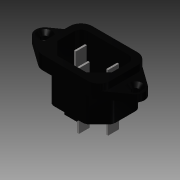
# Autodesk Inventor part: PowerSocket
Saved by Autodesk Inventor 2016 (Build 200138000, 138)
## iProperties
Category: Electronics
Created: 2014-09-28
Part Number: PowerSocket
Material: ABS Plastic
Document SubType Name: Modeling
Designer: Jack
Density: 1.06 g/cm^3
Appearance: Smooth - Black
Mass: 5.27757 g
Surface Area: 54.3399 cm^2
Volume: 4.97884 cm^3
Author: Jack
Title: Power Socket
Autodesk Inventor part; units mm, degrees
ref_plane "YZ Plane" through (0, 0, 0) normal (1, 0, 0) x (0, 1, 0)
ref_plane "XZ Plane" through (0, 0, 0) normal (0, 1, 0) x (-1, 0, 0)
ref_plane "XY Plane" through (0, 0, 0) normal (0, 0, 1) x (1, 0, 0)
sketch "Sketch1" plane through (0, 0, 0) normal (0, 0, 1) x (1, 0, 0)
  circle A0 centre (0, 0) radius 1.6
  circle A1 centre (40, 0) radius 1.6
  circle A2 centre (0, 0) radius 4
  circle A3 centre (40, 0) radius 4
  line L0 (8.5, 11) -> (31.5, 11)
  line L1 (8.5, -11) -> (31.5, -11)
  line L2 (8.5, 11) -> (-2.3275, 3.2531)
  line L3 (-2.3275, -3.2531) -> (8.5, -11)
  line L4 (31.5, -11) -> (42.3275, -3.2531)
  line L5 (42.3275, 3.2531) -> (31.5, 11)
  dimension "d0" = 3.2
  dimension "d2" = 40
  dimension "d3" = 8
  dimension "d5" = 23
  dimension "d6" = 11
  dimension "d7" = 11
  dimension "d8" = 8.5
  constraints: 12 end point, 4 centre point, 4 point on circle, 4 tangent, 3 coincident, 2 equal radius, 2 horizontal, 1 horizontal alignment, 1 parallel, 1 vertical alignment
  measures "d0" diameter of A0
  measures "d2" distance of point (0, 0) A1.centre
  measures "d3" diameter of A2
  measures "d5" distance of L0.start L0.end
  measures "d6" distance from line of point (0, 0) L0
  measures "d7" distance from line of point (0, 0) L1
  measures "d8" horizontal distance of point (0, 0) L0.start
extrude "Extrusion1" add sketch "Sketch1" along normal blind 3.1
sketch "Sketch2" plane through (0, 0, 3.1) normal (0, 0, 1) x (1, 0, 0)
  line L0 (8.5, -11) -> (31.5, -11) projected
  line L1 (31.5, 11) -> (8.5, 11) projected
  line L2 (5, -11) -> (5, 11)
  line L3 (5, 11) -> (35, 11)
  line L4 (35, 11) -> (35, -11)
  line L5 (35, -11) -> (5, -11)
  dimension "d11" = 30
  dimension "d12" = 3.5
  constraints: 8 end point, 2 collinear, 2 perpendicular, 1 point on line, 1 vertical
  measures "d11" distance of L2.end L3.end
  measures "d12" distance from line of L1.end L2
extrude "Extrusion2" add sketch "Sketch2" along normal blind 2.8
fillet "Fillet1" radius 5 4 edges at (5, -11, 4.5) (5, 11, 4.5) (35, 11, 4.5) (35, -11, 4.5)
fillet "Fillet2" radius 5 4 edges at (31.5, 11, 1.55) (8.5, 11, 1.55) (8.5, -11, 1.55) (31.5, -11, 1.55)
sketch "Sketch3" plane through (0, 0, 0) normal (0, 0, -1) x (-1, 0, 0)
  circle A0 centre (-40, 0) radius 1.6 projected
  line L0 (-29.8955, 11) -> (-10.1045, 11) projected
  line L1 (-33.5, 9.5) -> (-6.5, 9.5)
  line L2 (-6.5, 9.5) -> (-6.5, -9.5)
  line L3 (-6.5, -9.5) -> (-33.5, -9.5)
  line L4 (-33.5, -9.5) -> (-33.5, 9.5)
  dimension "d17" = 27
  dimension "d18" = 19
  dimension "d19" = 6.5
  dimension "d20" = 1.5
  constraints: 8 end point, 2 parallel, 1 horizontal, 1 perpendicular
  measures "d17" distance of L2.end L3.end
  measures "d18" distance of L1.end L2.end
  measures "d19" distance from line of A0.centre L4
  measures "d20" distance between parallel lines of L0 L1
extrude "Extrusion3" add sketch "Sketch3" along normal blind 12.7 contours L1 L2 L3 L4
chamfer "Chamfer1" distance 6 angle 45 2 edges at (33.5, -9.5, -6.35) (6.5, -9.5, -6.35)
fillet "Fillet3" radius 3 6 edges at (33.5, 9.5, -6.35) (6.5, 9.5, -6.35) (33.5, -3.5, -6.35) (27.5, -9.5, -6.35) (12.5, -9.5, -6.35) (6.5, -3.5, -6.35)
sketch "Sketch4" plane through (0, 0, -12.7) normal (0, 0, -1) x (-1, 0, 0)
  line L0 (-6.5, -2.2574) -> (-6.5, 6.5) projected
  line L1 (-9.5, 9.5) -> (-30.5, 9.5) projected
  line L2 (-33.5, 6.5) -> (-33.5, -2.2574) projected
  line L3 (-26.2574, -9.5) -> (-13.7426, -9.5) projected
  line L4 (-15.6, 8.6) -> (-10.2, 8.6)
  line L5 (-10.2, 8.6) -> (-10.2, -2.8)
  line L6 (-10.2, -2.8) -> (-15.6, -2.8)
  line L7 (-15.6, -2.8) -> (-15.6, 8.6)
  line L8 (-22.7, 2.8) -> (-17.3, 2.8)
  line L9 (-17.3, 2.8) -> (-17.3, -8.6)
  line L10 (-17.3, -8.6) -> (-22.7, -8.6)
  line L11 (-22.7, -8.6) -> (-22.7, 2.8)
  line L12 (-24.4, -2.8) -> (-29.8, -2.8)
  line L13 (-29.8, -2.8) -> (-29.8, 8.6)
  line L14 (-29.8, 8.6) -> (-24.4, 8.6)
  line L15 (-24.4, 8.6) -> (-24.4, -2.8)
  point P0 (0, 0)
  dimension "d27" = 5.4
  dimension "d28" = 11.4
  dimension "d29" = 3.7
  dimension "d30" = 3.7
  dimension "d31" = 1.7
  dimension "d32" = 0.9
  dimension "d33" = 0.9
  dimension "d34" = 0.9
  constraints: 24 end point, 6 parallel, 4 equal length, 3 horizontal, 3 perpendicular
  measures "d27" distance of L5.end L6.end
  measures "d28" distance of L4.end L5.end
  measures "d29" distance between parallel lines of L0 L5
  measures "d30" distance between parallel lines of L2 L13
  measures "d31" distance between parallel lines of L15 L11
  measures "d32" distance between parallel lines of L3 L10
  measures "d33" distance between parallel lines of L1 L14
  measures "d34" distance between parallel lines of L1 L4
extrude "Extrusion4" add sketch "Sketch4" along normal blind 1.8
sketch "Sketch5" plane through (0, 0, -14.5) normal (0, 0, -1) x (-1, 0, 0)
  line L0 (-24.4, -2.8) -> (-24.4, 8.6) projected
  line L1 (-24.4, 8.6) -> (-29.8, 8.6) projected
  line L2 (-17.3, 2.8) -> (-22.7, 2.8) projected
  line L3 (-22.7, 2.8) -> (-22.7, -8.6) projected
  line L4 (-22.7, -8.6) -> (-17.3, -8.6) projected
  line L5 (-17.3, -8.6) -> (-17.3, 2.8) projected
  line L6 (-10.2, 8.6) -> (-15.6, 8.6) projected
  line L7 (-15.6, 8.6) -> (-15.6, -2.8) projected
  line L8 (-15.6, -2.8) -> (-10.2, -2.8) projected
  line L9 (-10.2, -2.8) -> (-10.2, 8.6) projected
  line L10 (-27.5, 5.3) -> (-26.7, 5.3)
  line L11 (-26.7, 5.3) -> (-26.7, 0.5)
  line L12 (-26.7, 0.5) -> (-27.5, 0.5)
  line L13 (-27.5, 0.5) -> (-27.5, 5.3)
  line L14 (-13.3, 5.3) -> (-12.5, 5.3)
  line L15 (-12.5, 5.3) -> (-12.5, 0.5)
  line L16 (-12.5, 0.5) -> (-13.3, 0.5)
  line L17 (-13.3, 0.5) -> (-13.3, 5.3)
  line L18 (-20.4, -0.5) -> (-19.6, -0.5)
  line L19 (-19.6, -0.5) -> (-19.6, -5.3)
  line L20 (-19.6, -5.3) -> (-20.4, -5.3)
  line L21 (-20.4, -5.3) -> (-20.4, -0.5)
  point P0 (0, 0)
  dimension "d37" = 0.8
  dimension "d38" = 4.8
  dimension "d39" = 2.3
  dimension "d40" = 2.3
  dimension "d41" = 2.3
  dimension "d42" = 3.3
  dimension "d43" = 3.3
  constraints: 24 end point, 6 parallel, 4 equal length, 3 horizontal, 3 perpendicular, 1 horizontal alignment
  measures "d37" distance of L11.end L12.end
  measures "d38" distance of L10.end L11.end
  measures "d39" distance between parallel lines of L0 L11
  measures "d40" distance between parallel lines of L7 L17
  measures "d41" distance between parallel lines of L5 L19
  measures "d42" distance between parallel lines of L2 L18
  measures "d43" distance between parallel lines of L1 L10
extrude "Extrusion5" add sketch "Sketch5" along normal blind 7.5 contours L10 L11 L12 L13 | L14 L15 L16 L17 | L18 L19 L20 L21
sketch "Sketch6" plane through (0, 0, 5.9) normal (0, 0, 1) x (1, 0, 0)
  line L0 (30, 11) -> (10, 11) projected
  line L1 (5, 6) -> (5, -6) projected
  line L2 (8, 8) -> (32, 8)
  line L3 (32, 8) -> (32, -2.5)
  line L4 (26.5, -8) -> (13.5, -8)
  line L5 (8, -2.5) -> (8, 8)
  line L6 (8, -2.5) -> (13.5, -8)
  line L7 (32, -2.5) -> (26.5, -8)
  point P0 (0, 0)
  point P1 (32, -8)
  point P2 (8, -8)
  dimension "d46" = 24
  dimension "d47" = 16
  dimension "d48" = 3
  dimension "d49" = 3
  dimension "d50" = 5.5
  dimension "d51" = 5.5
  dimension "d52" = 5.5
  dimension "d53" = 5.5
  constraints: 12 end point, 4 point on line, 2 parallel, 1 horizontal, 1 perpendicular
  measures "d46" distance of point (32, -8) point (8, -8)
  measures "d47" distance of L2.end point (32, -8)
  measures "d48" distance between parallel lines of L1 L5
  measures "d49" distance between parallel lines of L0 L2
  measures "d50" distance of L5.start point (8, -8)
  measures "d51" distance of L4.end point (8, -8)
  measures "d52" distance of L3.end point (32, -8)
  measures "d53" distance of L4.start point (32, -8)
extrude "Extrusion6" cut sketch "Sketch6" against normal blind 16.8
fillet "Fillet4" radius 3 2 edges at (8, 8, -2.5) (32, 8, -2.5)
sketch "Sketch7" plane through (0, 0, -10.9) normal (0, 0, 1) x (1, 0, 0)
  line L0 (12.5, 5.3) -> (13.3, 5.3) projected
  line L1 (13.3, 5.3) -> (13.3, 0.5) projected
  line L2 (13.3, 0.5) -> (12.5, 0.5) projected
  line L3 (12.5, 0.5) -> (12.5, 5.3) projected
  line L4 (26.7, 5.3) -> (27.5, 5.3) projected
  line L5 (27.5, 5.3) -> (27.5, 0.5) projected
  line L6 (27.5, 0.5) -> (26.7, 0.5) projected
  line L7 (26.7, 0.5) -> (26.7, 5.3) projected
  line L8 (19.6, -0.5) -> (20.4, -0.5) projected
  line L9 (20.4, -0.5) -> (20.4, -5.3) projected
  line L10 (20.4, -5.3) -> (19.6, -5.3) projected
  line L11 (19.6, -5.3) -> (19.6, -0.5) projected
  point P0 (0, 0)
extrude "Extrusion7" add sketch "Sketch7" along normal blind 14
chamfer "Chamfer2" distance 1.5 angle 45 2 edges at (-1.6, 0, 3.1) (38.4, 0, 3.1)
equation "\"d51\" = d50"
equation "\"d52\" = d50"
equation "\"d53\" = d52"
body "Solid1"
